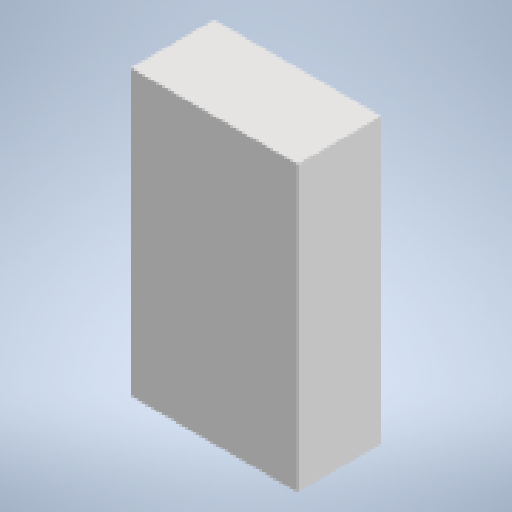
# Autodesk Inventor part: КонтроллерСпинер
Saved by Autodesk Inventor 2024.2 (Build 282272000, 272)
## iProperties
Created: 2025-03-13
Part Number: КонтроллерСпинер
Material: Пластик АБС
Document SubType Name: Modeling
Designer: Timofey
Density: 1.06 g/cm^3
Appearance: Гладкий — белый
Author: Timofey
Autodesk Inventor part; units mm, degrees
ref_plane "YZ Plane" through (0, 0, 0) normal (1, 0, 0) x (0, 1, 0)
ref_plane "XZ Plane" through (0, 0, 0) normal (0, 1, 0) x (-1, 0, 0)
ref_plane "XY Plane" through (0, 0, 0) normal (0, 0, 1) x (1, 0, 0)
sketch "Эскиз1" plane through (0, 0, 0) normal (1, 0, 0) x (0, 1, 0)
  line L0 (0, 0) -> (170, 0)
  line L1 (170, 0) -> (170, 50)
  line L2 (170, 50) -> (0, 50)
  line L3 (0, 50) -> (0, 0)
  dimension "d0" = 170
  dimension "d1" = 50
  constraints: 8 end point, 2 parallel, 1 horizontal, 1 perpendicular
  measures "d0" distance of L2.end L1.end
  measures "d1" distance of L1.end L0.end
extrude "Выдавливание1" add sketch "Эскиз1" along normal blind 100
